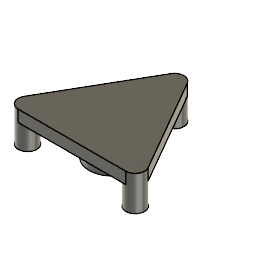
bearing rotor v3 (Autodesk Fusion 360 design; units mm, degrees)
part number: 2026-04-22-23-42-39-207
Autodesk Fusion 360 part; units mm, degrees
sketch "Sketch1" plane through (0, 0, 0) normal (0, 0, 1) x (1, 0, 0)
  circle A0 centre (0, 0) radius 21.59 construction
  line L0 (0, 27.546) -> (0, -31.973) construction
  line L1 (-40.4824, 0) -> (36.5438, 0) construction
  line L2 (0, 1.75) -> (0, 22.5)
  line L3 (1.75, 0) -> (22.5, 0)
  line L4 (-2, 1.5) -> (2, 1.5)
  line L5 (-2, -1.5) -> (2, -1.5)
  circle A1 centre (0, 0) radius 5.08
  arc A2 (-2, 1.5) -> (-2, -1.5) centre (0, 0) ccw
  arc A3 (2, -1.5) -> (2, 1.5) centre (0, 0) ccw
  circle A4 centre (0, 13.566) radius 6.5 construction
  circle A5 centre (0, 13.566) radius 2.05
  line L6 (7.62, 20.066) -> (-7.158, 20.066) construction
  line L7 (-11.43, 21.59) -> (19.6746, 21.59) construction
  dimension "d1" = 43.18
  dimension "d3" = 5
  dimension "d4" = 3
  dimension "d5" = 10.16
  dimension "d6" = 2.5
  dimension "d7" = 13
  dimension "d8" = 4.1
  dimension "d18" = 1.524
  constraint coincident A0.centre A1.centre
  constraint vertical L0
  constraint horizontal L1
  constraint collinear L0 L2
  constraint collinear L1 L3
  constraint concentric A0 A2
  constraint perpendicular L0 L4
  constraint perpendicular L0 L5
  constraint symmetric L1 L4 L5
  constraint concentric A0 A1
  constraint concentric A2 A3
  constraint coincident L0 A4.centre
  constraint concentric A4 A5
  constraint horizontal L6
  constraint horizontal L7
  constraint tangent A4 L6
  constraint tangent A0 L7
  measures "d1" diameter of A0
  measures "d3" diameter of A2
  measures "d4" distance of L4 L5
  measures "d5" diameter of A1
  measures "d6" radius of A3
  measures "d7" diameter of A4
  measures "d8" diameter of A5
  measures "d18" distance of L6 L7
extrude "Extrude1" add sketch "Sketch1" along normal blind 5.08 makes body 1 at (2.0475, 13.4638, 3.3867) makes body 2 at (5.0548, -0.5058, 1.6933)
pattern_circular "C-Pattern4" count 3 over 360 about axis through (0, 0, 1.75) along (0, 0, 1) of bodies 1 makes body 3 at (-12.6837, -4.9588, 3.3867) makes body 4 at (10.6363, -8.5051, 3.3867)
sketch "Sketch3" plane through (0, 0, 5.08) normal (0, 0, 1) x (-1, 0, 0)
  arc A0 (2, -1.5) -> (2, 1.5) centre (0, 0) ccw
  line L0 (2, -1.5) -> (-2, -1.5)
  arc A1 (-2, 1.5) -> (-2, -1.5) centre (0, 0) ccw
  line L1 (-2, 1.5) -> (2, 1.5)
  circle A2 centre (0, 0) radius 5.08
  line L2 (13.5239, 5.758) -> (1.7754, -14.591)
  line L3 (-1.7754, -14.591) -> (-13.5239, 5.758)
  line L4 (11.7485, 8.833) -> (-11.7485, 8.833)
  circle A3 centre (11.7485, 6.783) radius 2.05
  circle A4 centre (0, -13.566) radius 2.05
  circle A5 centre (-11.7485, 6.783) radius 2.05
  constraint horizontal L4
  constraint coincident L2.start A3
  constraint coincident L2.end A4
  constraint coincident L3.start A4
  constraint coincident L3.end A5
  constraint coincident L4.end A5
  constraint coincident L4.start A3
  constraint tangent L3 A4
  constraint tangent L2 A4
  constraint tangent L3 A5
  constraint tangent L2 A3
  constraint tangent L4 A3
extrude "Extrude4" add sketch "Sketch3" along normal blind 2.54 contours A0 L0 A1 L1 | A2 | L2 L3 L4 A3 A4 A5 | A3 | A4 | A5 bodies 1 2 3 4
